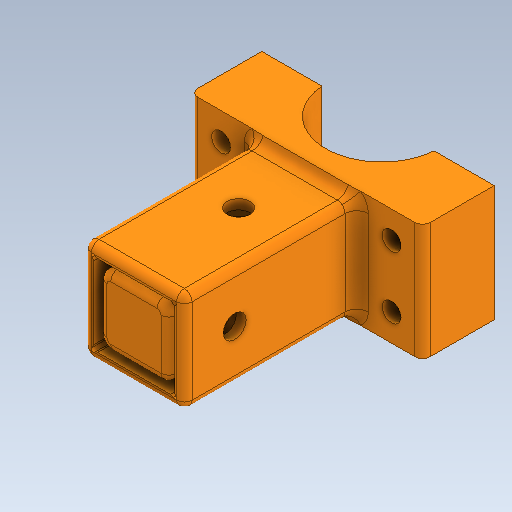
# Autodesk Inventor part: 2_Connettore_inf_sup
Saved by Autodesk Inventor 2020.2 (Build 242310000, 310)
## iProperties
Created: 2019-10-11
Part Number: 2_Connettore_inf_sup
Material: PLA(Stampato)(D0,646)
Document SubType Name: Modeling
Designer: socci
Density: 0.646 g/cm^3
Appearance: Arancione
Mass: 30.0332 g
Surface Area: 186.564 cm^2
Volume: 46.491 cm^3
Author: socci
Autodesk Inventor part; units mm, degrees
note: some values were not read from the file. Chosen so that the rebuilt part matches the saved one: direction of "Foro8"; direction of "Foro9"; edges of "Raccordo7".
ref_plane "YZ Plane" through (0, 0, 0) normal (1, 0, 0) x (0, 1, 0)
ref_plane "XZ Plane" through (0, 0, 0) normal (0, 1, 0) x (-1, 0, 0)
ref_plane "XY Plane" through (0, 0, 0) normal (0, 0, 1) x (1, 0, 0)
sketch "Schizzo1" plane through (0, 0, 0) normal (0, 0, 1) x (1, 0, 0)
  line L0 (7, -9) -> (-6, -9)
  line L1 (-9, -6) -> (-9, 6)
  line L2 (-6, 9) -> (6, 9)
  line L3 (9, 6) -> (9, -7)
  arc A0 (7, -9) -> (9, -7) centre (7, -7) ccw
  arc A1 (-9, -6) -> (-6, -9) centre (-6, -6) ccw
  arc A2 (-6, 9) -> (-9, 6) centre (-6, 6) ccw
  arc A3 (9, 6) -> (6, 9) centre (6, 6) ccw
  point P0 (0, 0)
  point P1 (0, 0)
  point P2 (9, -9)
  point P3 (-9, -9)
  point P4 (-9, 9)
  point P5 (9, 9)
  dimension "d0" = 18
  dimension "d44" = 2
  dimension "d45" = 3
  constraints: 8 end point, 8 point on circle, 8 point on line, 8 tangent, 4 centre point, 2 equal radius, 1 coincident, 9 other
  measures "d0" distance of point (-9, 9) point (9, 9)
  measures "d44" radius of A0
  measures "d45" radius of A1
extrude "Estrusione1" add sketch "Schizzo1" along normal blind 40
sketch "Schizzo2" plane through (0, 0, 0) normal (0, 0, -1) x (-1, 0, 0)
  line L0 (11, -13) -> (-11, -13)
  line L1 (-13, -11) -> (-13, 11)
  line L2 (-11, 13) -> (11, 13)
  line L3 (13, 11) -> (13, -11)
  line L4 (13, -13) -> (-13, 13) construction
  line L5 (-13, -13) -> (13, 13) construction
  arc A0 (13, 11) -> (11, 13) centre (11, 11) ccw
  arc A1 (11, -13) -> (13, -11) centre (11, -11) ccw
  arc A2 (-13, -11) -> (-11, -13) centre (-11, -11) ccw
  arc A3 (-11, 13) -> (-13, 11) centre (-11, 11) ccw
  point P0 (0, 0)
  dimension "d3" = 26
  dimension "d4" = 26
  dimension "d145" = 2
  constraints: 12 end point, 8 point on circle, 8 point on line, 8 tangent, 4 centre point, 3 equal radius, 3 midpoint, 2 parallel, 1 horizontal, 1 perpendicular
  measures "d3" distance of L4.start L5.start
  measures "d4" distance of L5.start L4.end
  measures "d145" radius of A0
extrude "Estrusione2" add sketch "Schizzo2" along normal blind 4.5
sketch "Schizzo12" plane through (0, 0, 0) normal (0, 0, 1) x (1, 0, 0)
  line L0 (-13, -11) -> (-13, 11)
  line L1 (-11, 13) -> (11, 13)
  line L2 (13, 11) -> (13, -11)
  line L3 (11, -13) -> (-11, -13)
  arc A0 (13, 11) -> (11, 13) centre (11, 11) ccw
  arc A1 (11, -13) -> (13, -11) centre (11, -11) ccw
  arc A2 (-13, -11) -> (-11, -13) centre (-11, -11) ccw
  arc A3 (-11, 13) -> (-13, 11) centre (-11, 11) ccw
  line L4 (-10.5, -9.382) -> (-10.5, 9.382)
  line L5 (-9.382, -10.5) -> (9.382, -10.5)
  line L6 (10.5, -9.382) -> (10.5, 9.382)
  line L7 (9.382, 10.5) -> (-9.382, 10.5)
  arc A4 (-10.1273, 10.8333) -> (-10.8333, 10.1273) centre (-10.5, 10.5) ccw
  arc A5 (-10.8333, -10.1273) -> (-10.1273, -10.8333) centre (-10.5, -10.5) ccw
  arc A6 (10.1273, -10.8333) -> (10.8333, -10.1273) centre (10.5, -10.5) ccw
  arc A7 (10.8333, 10.1273) -> (10.1273, 10.8333) centre (10.5, 10.5) ccw
  arc A8 (10.8333, 10.1273) -> (10.5, 9.382) centre (11.5, 9.382) ccw
  arc A9 (9.382, 10.5) -> (10.1273, 10.8333) centre (9.382, 11.5) ccw
  arc A10 (10.5, -9.382) -> (10.8333, -10.1273) centre (11.5, -9.382) ccw
  arc A11 (10.1273, -10.8333) -> (9.382, -10.5) centre (9.382, -11.5) ccw
  arc A12 (-9.382, -10.5) -> (-10.1273, -10.8333) centre (-9.382, -11.5) ccw
  arc A13 (-10.8333, -10.1273) -> (-10.5, -9.382) centre (-11.5, -9.382) ccw
  arc A14 (-10.1273, 10.8333) -> (-9.382, 10.5) centre (-9.382, 11.5) ccw
  arc A15 (-10.5, 9.382) -> (-10.8333, 10.1273) centre (-11.5, 9.382) ccw
  point P0 (0, 0)
  point P1 (0, 0)
  point P2 (-10.5, 10.5)
  point P3 (10.5, -10.5)
  point P4 (0, 0)
  point P5 (-13, -13)
  point P6 (-13, 13)
  point P7 (13, 13)
  point P8 (13, -13)
  point P9 (-10.5, -10)
  point P10 (-10.5, 10)
  point P11 (-10, -10.5)
  point P12 (10, -10.5)
  point P13 (10.5, -10)
  point P14 (10.5, 10)
  point P15 (10, 10.5)
  point P16 (-10, 10.5)
  point P17 (-10, 10.5)
  dimension "d110" = 21
  dimension "d111" = 26
  dimension "d180" = 1
  constraints: 40 point on circle, 24 tangent, 16 centre point, 16 end point, 16 point on line, 8 equal radius, 2 coincident, 2 vertical, 1 horizontal, 14 other
  measures "d110" distance of point (10.5, -10.5) point (-10.5, -10.5)
  measures "d111" distance of point (13, -13) point (-13, -13)
  measures "d180" radius of A8
extrude "Estrusione6" add sketch "Schizzo12" along normal blind 40
fillet "Raccordo3" radius 2 1 edges at (0, -13, 40)
sketch "Schizzo13" plane through (-11, -13, 0) normal (0, -1, 0) x (1, 0, 0)
  line L0 (11, 0) -> (11, 13)
  line L1 (11, 0) -> (24, 0) construction
  dimension "d118" = 13
  dimension "d119" = 90
  constraints: 4 end point, 1 horizontal, 1 perpendicular, 1 vertical
  measures "d118" distance of L0.start L0.end
  measures "d119" angle of L1 L0
hole "Foro8" at (0, -13, 13) direction (0, 1, 0) diameter 5.9 depth 26 clearance for "Vite a testa esagonale" size "M5" standard "ANSI - Profilo M Metrico"
sketch "Schizzo14" plane through (13, -11, 0) normal (1, 0, 0) x (0, 0, -1)
  line L0 (0, 11) -> (-27, 11)
  dimension "d127" = 27
  constraints: 2 end point, 1 horizontal
  measures "d127" distance of L0.start L0.end
hole "Foro9" at (13, 0, 27) direction (-1, 0, 0) diameter 5.9 depth 26 clearance for "Vite a testa esagonale" size "M5" standard "ANSI - Profilo M Metrico"
sketch "Schizzo17" plane through (0, 0, -4.5) normal (0, 0, -1) x (-1, 0, 0)
  line L0 (30, -15) -> (-30, -15)
  line L1 (-30, -15) -> (-30, 15)
  line L2 (-30, 15) -> (30, 15)
  line L3 (30, 15) -> (30, -15)
  line L4 (30, -15) -> (-30, 15) construction
  line L5 (-30, -15) -> (30, 15) construction
  point P0 (0, 0)
  point P1 (0, 0)
  point P2 (0, 0)
  dimension "d146" = 60
  dimension "d147" = 30
  constraints: 12 end point, 3 midpoint, 2 parallel, 1 coincident, 1 horizontal, 1 perpendicular
  measures "d146" distance of L0.start L0.end
  measures "d147" distance of L2.end L0.start
extrude "Estrusione7" add sketch "Schizzo17" along normal blind 18.5
sketch "Schizzo18" plane through (-30, -15, -4.5) normal (0, -1, 0) x (1, 0, 0)
  line L0 (30, 4.5) -> (30, -19.5)
  line L1 (30, 4.5) -> (54, 4.5) construction
  circle A0 centre (30, -19.5) radius 14.5
  dimension "d150" = 24
  dimension "d151" = 90
  dimension "d152" = 29
  constraints: 4 end point, 1 centre point, 1 coincident, 1 horizontal, 1 perpendicular, 1 vertical
  measures "d150" distance of L0.start L0.end
  measures "d151" angle of L0 L1
  measures "d152" diameter of A0
extrude "Estrusione8" cut sketch "Schizzo18" against normal blind 30
sketch "Schizzo19" plane through (0, 0, -4.5) normal (0, 0, 1) x (1, 0, 0)
  line L0 (30, -15) -> (-30, -15) projected
  line L1 (0, -15) -> (0, -8)
  line L2 (0, -15) -> (7, -15) construction
  line L3 (0, -8) -> (22, -8)
  line L4 (22, -8) -> (22, 8)
  line L5 (0, -8) -> (-22, -8)
  line L6 (-13, -11) -> (-13, 11) projected
  line L7 (0, -8) -> (22, -8) construction
  line L8 (-22, -8) -> (-22, 8)
  point P0 (0, 0)
  dimension "d155" = 7
  dimension "d156" = 90
  dimension "d157" = 22
  dimension "d158" = 90
  dimension "d159" = 16
  dimension "d160" = 90
  dimension "d161" = 22
  dimension "d162" = 180
  dimension "d163" = 16
  dimension "d164" = 90
  constraints: 14 end point, 4 perpendicular, 2 equal length, 2 horizontal, 1 midpoint, 1 vertical
  measures "d155" distance of L1.start L1.end
  measures "d156" angle of L2 L1
  measures "d157" distance of L1.end L3.end
  measures "d158" angle of L1 L3
  measures "d159" distance of L3.end L4.end
  measures "d160" angle of L4 L3
  measures "d161" distance of L1.end L5.end
  measures "d162" angle of L5 L7
  measures "d163" distance of L5.end L8.end
  measures "d164" angle of L5 L8
hole "Foro10" at (-22, -8, -4.5) at (-22, 8, -4.5) at (22, 8, -4.5) at (22, -8, -4.5) direction (0, 0, -1) diameter 4.9 end through all clearance for "Vite a testa piana" size "M4" standard "ANSI - Profilo M Metrico"
fillet "Raccordo5" radius 3 1 edges at (-13, 0, -4.5)
fillet "Raccordo6" radius 2 1 edges at (30, 0, -4.5)
fillet "Raccordo7" radius 2 1 edges at (-30, 0, -4.5)
fillet "Raccordo8" radius 2 1 edges at (0, 9, 40)
